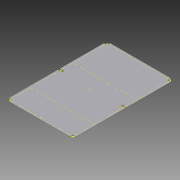
# Autodesk Inventor part: Bottom Sheet
Saved by Autodesk Inventor 2012 (Build 160160000, 160)
## iProperties
Created: 2011-10-20
Part Number: Bottom Sheet
Material: Aluminum-6061
Document SubType Name: Sheet Metal
Designer: Ian Walters
Density: 2.71 g/cm^3
Sheet Metal Rule: Default
Author: Ian Walters
Autodesk Inventor part; units mm, degrees
ref_plane "YZ Plane" through (0, 0, 0) normal (1, 0, 0) x (0, 1, 0)
ref_plane "XZ Plane" through (0, 0, 0) normal (0, 1, 0) x (-1, 0, 0)
ref_plane "XY Plane" through (0, 0, 0) normal (0, 0, 1) x (1, 0, 0)
derived "Cart Skeleton.ipt"
sketch "Sketch3" plane through (0, 0, 0) normal (0, 1, 0) x (-1, 0, 0)
  line L0 (-400.05, 603.25) -> (400.05, 603.25)
  line L1 (400.05, 603.25) -> (400.05, -603.25)
  line L2 (400.05, -603.25) -> (-400.05, -603.25)
  line L3 (-400.05, -603.25) -> (-400.05, 603.25)
  line L4 (400.05, 603.25) -> (361.95, 603.25)
  line L5 (361.95, 603.25) -> (361.95, 565.15)
  line L6 (361.95, 565.15) -> (400.05, 565.15)
  line L7 (400.05, 565.15) -> (400.05, 603.25)
  line L8 (-400.05, 603.25) -> (-361.95, 603.25)
  line L9 (-361.95, 603.25) -> (-361.95, 565.15)
  line L10 (-361.95, 565.15) -> (-400.05, 565.15)
  line L11 (-400.05, 565.15) -> (-400.05, 603.25)
  line L12 (-400.05, -603.25) -> (-361.95, -603.25)
  line L13 (-361.95, -603.25) -> (-361.95, -565.15)
  line L14 (-361.95, -565.15) -> (-400.05, -565.15)
  line L15 (-400.05, -565.15) -> (-400.05, -603.25)
  line L16 (400.05, -603.25) -> (361.95, -603.25)
  line L17 (361.95, -603.25) -> (361.95, -565.15)
  line L18 (361.95, -565.15) -> (400.05, -565.15)
  line L19 (400.05, -565.15) -> (400.05, -603.25)
  point P0 (0, 0)
  point P1 (-381, 584.2)
  point P2 (381, -584.2)
  dimension "d1" = 19.05
  dimension "d2" = 19.05
  dimension "d3" = 19.05
  dimension "d4" = 19.05
  dimension "d5" = 38.1
  measures "d1" horizontal distance of point (-381, 584.2) L0.start
  measures "d2" horizontal distance of L0.start point (-381, 584.2)
  measures "d3" horizontal distance of point (381, -584.2) L1.end
  measures "d4" horizontal distance of point (381, -584.2) L1.end
  measures "d5" distance of L9.end L10.end
extrude "Plate1" add sketch "Sketch3" along normal blind 3.175 contours L0 L5 L6 L1 L18 L17 L2 L13 L14 L3 L10 L9
sketch "Sketch2" plane through (0, 0, 0) normal (0, 1, 0) x (-1, 0, 0)
  line L0 (-381, 584.2) -> (381, 584.2)
  line L1 (381, 584.2) -> (381, -584.2)
  line L2 (381, -584.2) -> (-381, -584.2)
  line L3 (-381, -584.2) -> (-381, 584.2)
  line L4 (-381, 330.2) -> (381, 330.2)
  line L5 (-381, -177.8) -> (381, -177.8)
  point P0 (0, 0)
  point P1 (-381, 0)
  point P2 (0, 584.2)
  point P3 (-361.95, -28.5496)
  point P4 (361.95, -28.5496)
sketch "Sketch4" plane through (0, 0, 0) normal (0, -1, 0) x (1, 0, 0)
  line L0 (-361.95, 603.25) -> (-361.95, 565.15) projected
  line L1 (381, 584.2) -> (-381, 584.2) projected
  line L2 (381, 330.2) -> (-381, 330.2) projected
  line L3 (381, -177.8) -> (-381, -177.8) projected
  line L4 (-381, -584.2) -> (381, -584.2) projected
  circle A0 centre (-330.2, 584.2) radius 2.3813
  circle A1 centre (-330.2, 330.2) radius 2.3813
  circle A2 centre (-330.2, -177.8) radius 2.3813
  circle A3 centre (-330.2, -584.2) radius 2.3813
  point P0 (0, 0)
  dimension "d7" = 4.7625
  dimension "d8" = 31.75
  constraints: 4 centre point, 4 point on line, 3 equal radius, 3 vertical alignment
  measures "d7" diameter of A0
  measures "d8" distance from line of L0 A0.centre
extrude "Cut1" cut sketch "Sketch4" against normal blind 3.175
pattern_linear "Rectangular Pattern1" count 27 spacing 25.4 along (1, 0, 0) of "Cut1"
sketch "Sketch5" plane through (0, 0, 0) normal (0, -1, 0) x (1, 0, 0)
  line L0 (400.05, 565.15) -> (400.05, -565.15) projected
  line L1 (-400.05, -565.15) -> (-400.05, 565.15) projected
  line L2 (-400.05, -15.8496) -> (-349.25, -15.8496)
  line L3 (-349.25, -15.8496) -> (-349.25, -41.2496)
  line L4 (-349.25, -41.2496) -> (-400.05, -41.2496)
  line L5 (-400.05, -41.2496) -> (-400.05, -15.8496)
  line L6 (400.05, -41.2496) -> (349.25, -41.2496)
  line L7 (349.25, -41.2496) -> (349.25, -15.8496)
  line L8 (349.25, -15.8496) -> (400.05, -15.8496)
  line L9 (400.05, -15.8496) -> (400.05, -41.2496)
  point P0 (0, 0)
  point P1 (-361.95, -28.5496)
  point P2 (-374.65, -15.8496)
  point P3 (-349.25, -28.5496)
  dimension "d14" = 25.4
  dimension "d15" = 12.7
  constraints: 16 end point, 4 parallel, 3 horizontal alignment, 2 horizontal, 2 midpoint, 2 perpendicular, 2 point on line, 1 collinear
  measures "d14" distance of L2.end L3.end
  measures "d15" distance from line of L3 point (-361.95, -28.55)
extrude "Cut2" cut sketch "Sketch5" against normal blind 3.175
equation "\"d2\" = d1"
equation "\"d3\" = d1"
equation "\"d4\" = d1"
equation "\"d5\" = 2 * d1"
equation "\"d9\" = Thickness"
equation "\"d16\" = Thickness"
equation "\"BendRadius\" = Thickness"
equation "\"BendReliefWidth\" = Thickness"
equation "\"BendReliefDepth\" = 0.5 * Thickness"
equation "\"CornerReliefSize\" = 4 * Thickness"
equation "\"MinimumRemnant\" = 2 * Thickness"
equation "\"TransitionRadius\" = BendRadius"
equation "\"JacobiRadiusSize\" = Thickness"
equation "\"GapSize\" = Thickness"
equation "\"d6\" = BendRadius"
equation "\"Thickness\" = 3.175"
body "Solid1"
